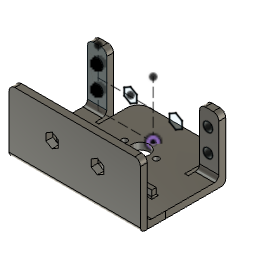
servo base stand v2 v6 (Autodesk Fusion 360 design; units mm, degrees)
Autodesk Fusion 360 part; units mm, degrees
sketch "Sketch1" plane through (0, 0, 0) normal (0, 0, 1) x (1, 0, 0)
  line L0 (-29, 18) -> (29, 18)
  line L1 (29, 18) -> (29, -18)
  line L2 (29, -18) -> (-29, -18)
  line L3 (-29, -18) -> (-29, 18)
  line L4 (-29, 18) -> (29, -18) construction
  line L5 (29, 18) -> (-29, -18) construction
  line L6 (29, 8.6) -> (-29, 8.6) construction
  line L7 (-29, -18) -> (-29, -26)
  line L8 (-29, -26) -> (29, -26)
  line L9 (29, -26) -> (29, -18)
  line L10 (29, -26) -> (29, -29)
  line L11 (29, -29) -> (-29, -29)
  line L12 (-29, -29) -> (-29, -26)
  line L13 (-29, 5.6) -> (-20.5, 5.6)
  line L14 (-20.5, 5.6) -> (-20.5, 8.6)
  line L15 (-20.5, 8.6) -> (-29, 8.6)
  line L16 (-20.5, 5.6) -> (-20.5, 0.6)
  line L17 (-20.5, 0.6) -> (-19, 0.6)
  line L18 (-19, 0.6) -> (-19, 8.6)
  line L19 (0, -29) -> (0, 18) construction
  line L20 (20.5, 8.6) -> (29, 8.6)
  line L21 (20.5, 5.6) -> (20.5, 8.6)
  line L22 (29, 5.6) -> (20.5, 5.6)
  line L23 (20.5, 5.6) -> (20.5, 0.6)
  line L24 (20.5, 0.6) -> (19, 0.6)
  line L25 (19, 0.6) -> (19, 8.6)
  circle A0 centre (0, 0) radius 4
  circle A1 centre (0, 0) radius 7 construction
  circle A2 centre (0, 7) radius 1.25
  circle A3 centre (-7, 0) radius 1.25
  circle A4 centre (0, -7) radius 1.25
  circle A5 centre (7, 0) radius 1.25
  line L26 (-19, 8.6) -> (-20.5, 8.6)
  line L27 (19, 8.6) -> (20.5, 8.6)
  line L28 (-19, 8.6) -> (-19, 18)
  line L29 (19, 8.6) -> (19, 18)
  line L30 (-21, -14) -> (-15, -14)
  line L31 (-15, -14) -> (-15, -16)
  line L32 (-15, -16) -> (-21, -16)
  line L33 (-21, -16) -> (-21, -14)
  line L34 (15, -14) -> (15, -16)
  line L35 (21, -16) -> (21, -14)
  line L36 (15, -16) -> (21, -16)
  line L37 (21, -14) -> (15, -14)
  line L38 (0, -7) -> (29, -7) construction
  circle A6 centre (0, -14) radius 4
  circle A7 centre (0, -21) radius 1.25
  circle A8 centre (7, -14) radius 1.25
  circle A9 centre (-7, -14) radius 1.25
  dimension "d4" = 36
  dimension "d5" = 58
  dimension "d9" = 26.6
  dimension "d11" = 8
  dimension "d12" = 8
  dimension "d13" = 3
  dimension "d14" = 3
  dimension "d16" = 8.5
  dimension "d17" = 3
  dimension "d18" = 1.5
  dimension "d19" = 8
  dimension "d22" = 8
  dimension "d23" = 14
  dimension "d24" = 2.5
  dimension "d26" = 360
  dimension "d56" = 2
  dimension "d57" = 6
  dimension "d58" = 8
  dimension "d59" = 2
  constraint horizontal L0
  constraint perpendicular L0 L1
  constraint parallel L0 L2
  constraint parallel L1 L3
  constraint coincident L4 A0.centre
  constraint coincident L5 A0.centre
  constraint coincident A0.centre A1.centre
  constraint coincident L1 L6.start
  constraint coincident L3 L6.end
  constraint perpendicular L3 L6
  constraint perpendicular L2 L7
  constraint perpendicular L7 L8
  constraint perpendicular L8 L10
  constraint perpendicular L10 L11
  constraint coincident L3 L13.start
  constraint perpendicular L3 L13
  constraint coincident L6 L14.end
  constraint perpendicular L6 L14
  constraint perpendicular L3 L15
  constraint perpendicular L13 L16
  constraint perpendicular L16 L17
  constraint coincident L6 L18.end
  constraint perpendicular L6 L18
  constraint midpoint L11 L19.start
  constraint midpoint L0 L19.end
  constraint symmetric L6.end L19 L6.start
  constraint symmetric L13.start L19 L22.start
  constraint symmetric L13.end L19 L21.start
  constraint symmetric L14.end L19 L20.start
  constraint symmetric L16.end L19 L23.end
  constraint symmetric L17.end L19 L24.end
  constraint symmetric L18.end L19 L25.end
  constraint coincident L19 A2.centre
  constraint coincident A1 A2.centre
  constraint coincident L0 L28.end
  constraint perpendicular L0 L28
  constraint coincident L0 L29.end
  constraint perpendicular L0 L29
  constraint horizontal L30
  constraint vertical L31
  constraint horizontal L32
  constraint vertical L33
  constraint symmetric L19 L30.start L35.end
  constraint symmetric L19 L30.end L34.start
  constraint symmetric L19 L31.end L34.end
  constraint symmetric L19 L32.end L35.start
  constraint coincident A4.centre L38.start
  constraint coincident L1 L38.end
  constraint tangent A1 L38
  constraint symmetric A0 L38 A6
  constraint symmetric A2 L38 A7
  constraint symmetric A3 L38 A9
  constraint symmetric A5 L38 A8
  measures "d4" distance of L0.end L1.end
  measures "d5" distance of L1.end L2.end
  measures "d9" distance of L2 L6
  measures "d11" distance of L2.end L7.end
  measures "d12" distance of L1.end L8.end
  measures "d13" distance of L7.end L11.end
  measures "d14" distance of L8.end L10.end
  measures "d16" distance of L13.start L13.end
  measures "d17" distance of L13.end L14.end
  measures "d18" distance of L16.end L17.end
  measures "d19" distance of L17.end L18.end
  measures "d22" diameter of A0
  measures "d23" diameter of A1
  measures "d24" diameter of A2
  measures "d56" distance of L30.start L32.end
  measures "d57" distance of L31.end L32.end
  measures "d58" distance of L3 L33
  measures "d59" distance of L2 L32
extrude "Extrude3" add sketch "Sketch1" against normal blind 3 contours L0 L1 L2 L3 L13 L16 L17 L18 L22 L23 L24 L25 L28 L29 | L3 L13 L14 L15 | L2 L7 L8 L9 | L1 L20 L21 L22 | L8 L10 L11 L12 | L30 L31 L32 L33 | L34 L35 L36 L37
extrude "Extrude4" add sketch "Sketch1" along normal blind 25 contours L3 L13 L14 L15 | L1 L20 L21 L22 | L8 L10 L11 L12
fillet "Fillet1" radius 2.5 6 edges at (29, -27.5, 25) (-29, -27.5, 25) (29, 7.1, 25) (-29, 7.1, 25) (-20.5, 7.1, 25) (20.5, 7.1, 25)
fillet "Fillet2" radius 5 2 edges at (19, 18, -1.5) (-19, 18, -1.5)
fillet "Fillet3" radius 2 6 edges at (0, -26, 0) (0, -29, -3) (24.75, 5.6, 0) (24.75, 8.6, -3) (-24.75, 8.6, -3) (-24.75, 5.6, 0)
fillet "Fillet3" radius 1 6 edges at (-19, 6.8, -3) (-17.5355, 16.5355, -3) (0, 18, -3) (17.5355, 16.5355, -3) (19, 10.8, -3) (19, 4.6, -3)
sketch "Sketch3" plane through (0, 5.6, 0) normal (0, -1, 0) x (1, 0, 0)
  line L0 (-29, 2) -> (-20.5, 2)
  line L1 (-20.5, 2) -> (-20.5, 22.5)
  arc A0 (-20.5, 22.5) -> (-23, 25) centre (-23, 22.5) ccw
  line L2 (-23, 25) -> (-26.5, 25)
  arc A1 (-26.5, 25) -> (-29, 22.5) centre (-26.5, 22.5) ccw
  line L3 (-29, 22.5) -> (-29, 2)
  line L4 (0, 0) -> (0, 25) construction
  line L5 (0, 0) -> (-24.25, 0) construction
  line L6 (-24.25, 0) -> (-24.25, 25) construction
  line L7 (-24.25, 12.5) -> (0, 12.5) construction
  circle A2 centre (-24.25, 8) radius 2
  circle A3 centre (-24.25, 18) radius 2
  line L8 (-7.25, 14.5877) -> (-10, 16.1754)
  line L9 (-10, 16.1754) -> (-12.75, 14.5877)
  line L10 (-12.75, 14.5877) -> (-12.75, 11.4123)
  line L11 (-12.75, 11.4123) -> (-10, 9.8246)
  line L12 (-10, 9.8246) -> (-7.25, 11.4123)
  line L13 (-7.25, 11.4123) -> (-7.25, 14.5877)
  circle A4 centre (24.25, 18) radius 2
  circle A5 centre (24.25, 8) radius 2
  line L14 (12.75, 11.4123) -> (10, 9.8246)
  line L15 (12.75, 14.5877) -> (12.75, 11.4123)
  line L16 (10, 16.1754) -> (12.75, 14.5877)
  line L17 (7.25, 14.5877) -> (10, 16.1754)
  line L18 (7.25, 11.4123) -> (7.25, 14.5877)
  line L19 (10, 9.8246) -> (7.25, 11.4123)
  point P0 (-10, 13)
  dimension "d49" = 25
  dimension "d50" = 24.25
  dimension "d51" = 25
  dimension "d52" = 4
  dimension "d53" = 4.5
  dimension "d54" = 10
  dimension "d55" = 4
  dimension "d64" = 2.75
  dimension "d65" = 0.5
  dimension "d66" = 14.25
  constraint coincident L4.start L5.start
  constraint vertical L4
  constraint perpendicular L4 L5
  constraint perpendicular L2 L6
  constraint midpoint L6 L7.start
  constraint midpoint L4 L7.end
  constraint coincident L6 A2.centre
  constraint coincident L6 A3.centre
  constraint vertical L10
  constraint symmetric L4 A2 A5
  constraint symmetric L4 A3 A4
  constraint symmetric L4 L8.start L17.start
  constraint symmetric L4 L8.end L16.start
  constraint symmetric L4 L9.end L15.start
  constraint symmetric L4 L10.end L14.start
  constraint symmetric L4 L11.end L14.end
  constraint symmetric L4 L12.end L18.start
  measures "d49" distance of L4.start L4.end
  measures "d50" distance of L4.start L5.end
  measures "d51" distance of L5.end L6.end
  measures "d52" diameter of A2
  measures "d53" distance of L7 A2.centre
  measures "d54" distance of A2.centre A3.centre
  measures "d55" diameter of A3
  measures "d64" distance of P0 L13
  measures "d65" distance of L7 P0
  measures "d66" distance of L6 P0
extrude "Extrude5" add sketch "Sketch1" along normal blind 3 contours L30 L31 L32 L33 | L34 L35 L36 L37
fillet "Fillet4" radius 0.5 8 edges at (18, -14, 0) (21, -15, 0) (18, -16, 0) (15, -15, 0) (-15, -15, 0) (-18, -14, 0) (-21, -15, 0) (-18, -16, 0)
extrude "Extrude6" cut sketch "Sketch3" against normal through all contours A2 | A3 | A4 | A5
extrude "Extrude7" cut sketch "Sketch3" along normal blind 42 contours L8 L9 L10 L11 L12 L13 | L14 L15 L16 L17 L18 L19
equation "thickness = 3 mm"
equation "base_width = 36 mm"
equation "base_length = 58 mm"
equation "d4 = base_width"
equation "d5 = base_length"
equation "d9 = servoHolder_height"
equation "servo_clearence = 8 mm"
equation "d11 = servo_clearence"
equation "d12 = servo_clearence"
equation "d13 = thickness"
equation "d14 = thickness"
equation "servoHolder_height = 26.6 mm"
equation "d17 = thickness"
equation "main_hole = 8 mm"
equation "titner_hole = 2.5 mm"
equation "d22 = main_hole"
equation "d24 = titner_hole"
equation "base_height = 25 mm"
equation "d32 = -thickness"
equation "d34 = base_height"
equation "d50 = ( 48.5 / 2 ) * 1 mm"
equation "d64 = ( 5.5 / 2 ) * 1 mm"
